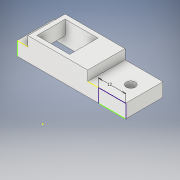
# Autodesk Inventor part: SG90 360 Degree Servo Holder
Saved by Autodesk Inventor 2019 (Build 230136000, 136)
## iProperties
Created: 2022-01-04
Part Number: SG90 360 Degree Servo Holder
Material: Generic
Description: STEP AP214
Document SubType Name: Modeling
Designer: Garrett Raker
Density: 1 g/cm^3
Appearance: Default
Sending System: SolidWorks 2020
Preprocessor: SwSTEP 2.0
Title: SG90 Servo.STEP
Revision Number: ANY
Autodesk Inventor part; units mm, degrees
ref_plane "YZ Plane" through (0, 0, 0) normal (1, 0, 0) x (0, 1, 0)
ref_plane "XZ Plane" through (0, 0, 0) normal (0, 1, 0) x (-1, 0, 0)
ref_plane "XY Plane" through (0, 0, 0) normal (0, 0, 1) x (1, 0, 0)
ref_plane "Work Plane1" through (14.1733, 21.9678, -54.6168) normal (0, 0, -1) x (-1, 0, 0)
sketch "Sketch1" plane through (14.1733, 21.9678, -54.6168) normal (0, 0, -1) x (-1, 0, 0)
  line L0 (-7.7, 2.5) -> (-8.55, 2.5) projected
  line L1 (-3.75, 6.7) -> (-3.75, 2.5) projected
  line L2 (-2.9, 6.8) -> (-3.65, 6.8) projected
  line L3 (4.25, 6.9) -> (4.25, 10.95) projected
  line L4 (-7.3526, 2.5) -> (-8.55, 2.5) projected
  line L5 (-3.75, 6.7) -> (-3.75, 2.5) projected
  line L6 (-8.55, 2.5) -> (-3.75, 2.5)
  line L7 (-3.75, 2.5) -> (-3.75, 6.8)
  line L8 (-3.75, 6.8) -> (4.15, 6.8)
  arc A0 (4.15, 6.8) -> (4.25, 6.9) centre (4.15, 6.9) ccw projected
  line L9 (-8.55, 2.5) -> (-8.55, -1.5)
  line L10 (23.55, 2.5) -> (23.55, 0) projected
  line L11 (23.55, 2.5) -> (23.55, -1.5)
  line L12 (23.55, 2.5) -> (18.75, 2.5)
  line L13 (4.25, 10.95) -> (18.75, 10.95)
  line L14 (-8.55, -1.5) -> (23.55, -1.5)
  line L15 (4.25, 10.95) -> (7.05, 10.95) projected
  line L16 (4.25, 6.9) -> (4.25, 10.95)
  arc A1 (4.15, 6.8) -> (4.25, 6.9) centre (4.15, 6.9) ccw
  line L17 (18.75, 10.95) -> (18.75, 2.5)
  point P0 (14.1733, -21.9678)
  point P1 (-8.55, 0)
  dimension "d1" = 4
  dimension "d2" = 4
  dimension "d3" = 4.8
  constraints: 20 end point, 3 perpendicular, 2 point on circle, 2 vertical, 1 centre point, 1 coincident, 1 collinear, 1 concentric, 1 horizontal, 1 point on line
  measures "d1" distance of L0.end L9.end
  measures "d2" distance of L10.start L11.end
  measures "d3" distance of L10.start L12.end
extrude "Extrusion1" add sketch "Sketch1" along normal mid plane 12.5
shell "Shell1" thickness 2 outward yes removed faces 1 at (1.3233, 20.4678, -56.7001)
sketch "Sketch2" plane through (14.1733, 21.9678, -62.8668) normal (0, 0, -1) x (-1, 0, 0)
  line L0 (-5.75, 8.8) -> (2.25, 8.8) projected
  line L1 (20.75, 12.95) -> (2.25, 12.95)
  line L2 (2.25, 12.95) -> (2.25, 8.8)
  line L3 (2.25, 8.8) -> (20.75, 8.8)
  line L4 (20.75, 8.8) -> (20.75, 12.95)
  point P0 (14.1733, -21.9678)
  point P1 (2.25, 12.95)
  constraints: 8 end point, 2 parallel, 1 horizontal, 1 perpendicular
extrude "Extrusion2" cut sketch "Sketch2" against normal up to surface (16.5 mm away)
sketch "Sketch3" plane through (14.1733, 21.9678, -46.3668) normal (0, 0, 1) x (1, 0, 0)
  line L0 (-25.55, 4.5) -> (-20.75, 4.5) projected
  line L1 (-25.55, -1.5) -> (-25.55, 4.5)
  line L2 (5.75, 4.5) -> (10.55, 4.5) projected
  line L3 (10.55, 4.5) -> (22.55, 4.5)
  line L4 (22.55, 4.5) -> (22.55, -1.5)
  line L5 (22.55, -1.5) -> (10.55, -1.5)
  line L6 (10.55, -1.5) -> (10.55, 4.5)
  point P0 (-14.1733, -21.9678)
  dimension "d21" = 12
  constraints: 10 end point, 2 parallel, 1 horizontal, 1 perpendicular
  measures "d21" distance of L2.end L3.end
extrude "Extrusion3" add sketch "Sketch3" against normal up to surface (16.5 mm away)
sketch "Sketch5" plane through (19.9233, 26.4678, -46.3668) normal (0, 1, 0) x (1, 0, 0)
  circle A0 centre (10.8, 8.25) radius 2
  line L0 (16.8, 0) -> (16.8, 16.5) projected
  line L1 (0, 16.5) -> (16.8, 16.5) projected
  point P0 (-19.9233, -46.3668)
  dimension "d22" = 4
  dimension "d23" = 6
  dimension "d25" = 8.25
  constraints: 1 centre point
  measures "d22" diameter of A0
  measures "d23" distance from line of L0 A0.centre
  measures "d25" distance from line of L1 A0.centre
extrude "Extrusion4" cut sketch "Sketch5" against normal through all
body "Solid1"
body "Solid3"
